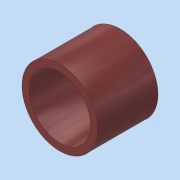
# Autodesk Inventor part: SleeveBearing.25inch
Saved by Autodesk Inventor 2017 (Build 210142000, 142)
## iProperties
Created: 2017-09-01
Part Number: SleeveBearing.25inch
Material: Bronze, Cast
Document SubType Name: Modeling
Designer: Derek Wider
Density: 8.87 g/cm^3
Appearance: Chestnut
Author: Derek Wider
Autodesk Inventor part; units mm, degrees
ref_plane "YZ Plane" through (0, 0, 0) normal (1, 0, 0) x (0, 1, 0)
ref_plane "XZ Plane" through (0, 0, 0) normal (0, 1, 0) x (-1, 0, 0)
ref_plane "XY Plane" through (0, 0, 0) normal (0, 0, 1) x (1, 0, 0)
sketch "Sketch1" plane through (0, 0, 0) normal (0, 0, 1) x (1, 0, 0)
  circle A0 centre (0, 0) radius 3.2258
  circle A1 centre (0, 0) radius 3.9688
  dimension "d0" = 7.9375
  dimension "d1" = 6.4516
  constraints: 2 centre point, 2 coincident
  measures "d0" diameter of A1
  measures "d1" diameter of A0
extrude "Extrusion1" add sketch "Sketch1" along normal blind 6.35
body "Solid1"
